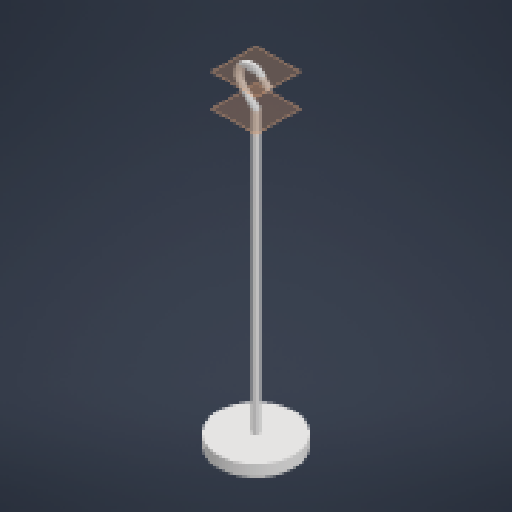
# Autodesk Inventor part: Long Hanging Mass
Saved by Autodesk Inventor 2023.1 (Build 271208000, 208)
## iProperties
Created: 2022-12-07
Part Number: Long Hanging Mass
Material: Generic
Document SubType Name: Modeling
Designer: aubrey-work
Density: 1 g/cm^3
Appearance: Default
Author: aubrey-work
Autodesk Inventor part; units mm, degrees
ref_plane "YZ Plane" through (0, 0, 0) normal (1, 0, 0) x (0, 1, 0)
ref_plane "XZ Plane" through (0, 0, 0) normal (0, 1, 0) x (-1, 0, 0)
ref_plane "XY Plane" through (0, 0, 0) normal (0, 0, 1) x (1, 0, 0)
sketch "Sketch1" plane through (0, 0, 0) normal (0, 1, 0) x (-1, 0, 0)
  circle A0 centre (0, 0) radius 19.05
  dimension "d0" = 38.1
  constraints: 1 centre point, 1 coincident
  measures "d0" diameter of A0
extrude "Extrusion1" add sketch "Sketch1" along normal mid plane 6.35
sketch "Sketch2" plane through (0, 0, 0) normal (0, 0, 1) x (1, 0, 0)
  line L0 (19.05, 3.175) -> (-19.05, 3.175) projected
  line L1 (0, 3.175) -> (0, 142.875)
  line L2 (0, 142.875) -> (-2.2451, 145.1201)
  line L3 (0, 142.875) -> (3.175, 142.875) construction
  circle A0 centre (-2.2451, 154.1003) radius 6.35 construction
  line L4 (-2.2451, 145.1201) -> (34.3651, 181.7303) construction
  line L5 (-2.2451, 145.1201) -> (-6.7352, 149.6102)
  line L6 (2.2451, 158.5904) -> (6.7352, 154.1003)
  arc A1 (2.2451, 158.5904) -> (-6.7352, 149.6102) centre (-2.2451, 154.1003) ccw
  point P0 (0, 0)
  dimension "d3" = 139.7
  dimension "d4" = 3.175
  dimension "d5" = 135
  dimension "d6" = 12.7
  dimension "d7" = 6.35
  dimension "d14" = 17.5753
  constraints: 12 end point, 5 tangent, 4 point on circle, 2 centre point, 1 equal length, 1 horizontal, 1 midpoint, 1 parallel, 1 perpendicular, 1 vertical
  measures "d3" distance of L1.start L1.end
  measures "d4" distance of L1.end L2.end
  measures "d5" angle of L3 L2
  measures "d6" diameter of A0
  measures "d7" distance of L6.start L6.end
sketch "Sketch3" plane through (0, 3.175, 0) normal (0, 1, 0) x (1, 0, 0)
  circle A0 centre (0, 0) radius 1.5875
  dimension "d8" = 3.175
  constraints: 1 centre point, 1 coincident
  measures "d8" diameter of A0
sweep "Sweep1" add profiles "Sketch3" path "Sketch2" path curves L1 L2 L5 A1 L6
chamfer "Chamfer1" distance 0.635 angle 45 1 edges at (19.05, -3.175, 0)
ref_plane "Work Plane2" through (0, 158.8628, 0) normal (0, 1, 0) x (-1, 0, 0)
ref_plane "Work Plane1" through (0, 142.875, 0) normal (0, 1, 0) x (-1, 0, 0)
sketch "Sketch4" plane through (0, 158.8628, 0) normal (0, 1, 0) x (-1, 0, 0)
  ellipse E0 centre (-2.2451, 0) end of major axis (-2.2451, -1.5875) minor radius 1.1225 projected
  ellipse E1 centre (6.7352, 0) end of major axis (6.7352, -1.5875) minor radius 1.1225 projected
  line L0 (-2.2451, 0) -> (6.7352, 0) construction
  line L1 (0.6576, 1.5875) -> (3.8326, 1.5875)
  line L2 (3.8326, 1.5875) -> (3.8326, -1.5875)
  line L3 (3.8326, -1.5875) -> (0.6576, -1.5875)
  line L4 (0.6576, -1.5875) -> (0.6576, 1.5875)
  line L5 (0.6576, 1.5875) -> (3.8326, -1.5875) construction
  line L6 (3.8326, 1.5875) -> (0.6576, -1.5875) construction
  point P0 (0, 0)
  point P1 (2.2451, 0)
  dimension "d8" = 3.175
  dimension "d16" = 3.175
  dimension "d17" = 3.175
  constraints: 14 end point, 3 midpoint, 2 horizontal, 2 parallel, 1 perpendicular, 2 other
  measures "d16" distance of L2.end L3.end
  measures "d17" distance of L1.end L2.end
extrude "Extrusion2" add sketch "Sketch4" along normal through all contours L1 L2 L3 L4
equation "\"d16\" = d8"
equation "\"d17\" = d8"
equation "\"d15\" = d14 - 0.5 * d8"
body "Solid1"
